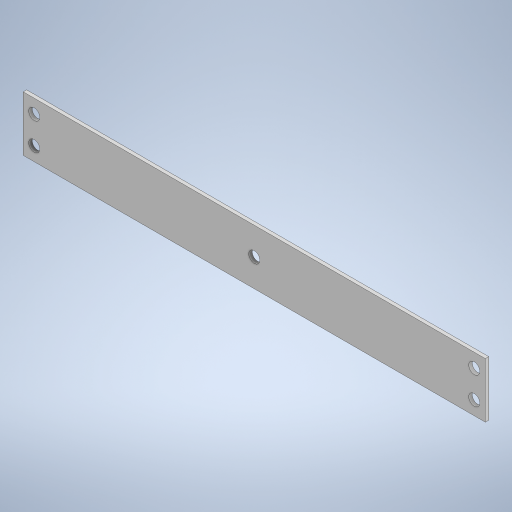
# Autodesk Inventor part: Intake Poly (Triball Holder)
Saved by Autodesk Inventor 2023 (Build 270158000, 158)
## iProperties
Created: 2024-02-16
Part Number: Intake Poly (Triball Holder)
Material: Generic
Document SubType Name: Modeling
Designer: Robodox
Density: 1 g/cm^3
Appearance: Default
Author: Robodox
Autodesk Inventor part; units mm, degrees
ref_plane "YZ Plane" through (0, 0, 0) normal (1, 0, 0) x (0, 1, 0)
ref_plane "XZ Plane" through (0, 0, 0) normal (0, 1, 0) x (-1, 0, 0)
ref_plane "XY Plane" through (0, 0, 0) normal (0, 0, 1) x (1, 0, 0)
sketch "Sketch1" plane through (0, 0, 0) normal (0, 0, 1) x (1, 0, 0)
  line L0 (-101.503, 53.7457) -> (111.857, 53.7457)
  line L1 (111.857, 53.7457) -> (111.857, 28.3457)
  line L2 (111.857, 28.3457) -> (-101.503, 28.3457)
  line L3 (-101.503, 28.3457) -> (-101.503, 53.7457)
  line L4 (-101.503, 53.7457) -> (-101.503, 47.3957)
  line L5 (-101.503, 47.3957) -> (-96.423, 47.3957)
  line L6 (-96.423, 47.3957) -> (-96.423, 53.7457)
  circle A0 centre (-96.423, 47.3957) radius 2.54
  line L7 (-96.423, 47.3957) -> (-96.423, 34.6957)
  circle A1 centre (-96.423, 34.6957) radius 2.54
  line L8 (-96.423, 47.3957) -> (106.777, 47.3957)
  circle A2 centre (106.777, 47.3957) radius 2.54
  line L9 (106.777, 47.3957) -> (106.777, 34.6957)
  circle A3 centre (106.777, 34.6957) radius 2.54
  line L10 (-96.423, 41.0457) -> (5.177, 41.0457)
  circle A4 centre (5.177, 41.0457) radius 2.54
  point P0 (0, 0)
  point P1 (-98.963, 47.3957)
  point P2 (-96.423, 49.9357)
  dimension "d0" = 213.36
  dimension "d1" = 25.4
  dimension "d2" = 6.35
  dimension "d3" = 5.08
  dimension "d4" = 5.08
  dimension "d5" = 12.7
  dimension "d6" = 5.08
  dimension "d7" = 203.2
  dimension "d8" = 5.08
  dimension "d9" = 12.7
  dimension "d10" = 5.08
  dimension "d11" = 5.08
  constraints: 22 end point, 5 centre point, 5 coincident, 4 perpendicular, 3 parallel, 2 horizontal, 2 point on line, 1 midpoint, 1 vertical
  measures "d0" distance of L0.start L0.end
  measures "d1" distance of L2.end L0.start
  measures "d2" distance of L0.start L4.end
  measures "d3" distance of L4.end L5.end
  measures "d4" diameter of A0
  measures "d5" distance of L7.start L7.end
  measures "d6" diameter of A1
  measures "d7" distance of L7.start L8.end
  measures "d8" diameter of A2
  measures "d9" distance of L9.start L9.end
  measures "d10" diameter of A3
  measures "d11" diameter of A4
extrude "Extrusion1" add sketch "Sketch1" along normal blind 1.5875 contours L0 L6 A0 L5 L3 | L0 L1 L2 L3 L5 A0 L6
body "Solid1"
